Autodesk Inventor part; units mm, degrees
(part 2 of 2)
  line L170 (-11.4491, 40.8252) -> (-11.4491, 40.6608)
  line L171 (-11.4491, 40.6608) -> (-13.491, 40.6608)
  line L172 (-13.491, 40.6608) -> (-13.491, 40.8252)
  spline S328 degree 2 poles (-13.491, 40.8252) (-13.2171, 40.8252) (-13.0627, 40.9098) knots 0 0 0 1 1 1
  spline S329 degree 2 poles (-13.0627, 40.9098) (-12.9731, 40.9547) (-12.8635, 41.2087) (-12.8635, 41.5922) knots 0 0 0 1 2 2 2
  line L173 (-12.8635, 41.5922) -> (-12.8635, 45.3225)
  spline S330 degree 2 poles (-12.8635, 45.3225) (-12.8635, 46.0247) (-12.9332, 46.3435) (-13.0727, 46.458) (-13.1872, 46.458) knots 0 0 0 1 2 3 3 3
  spline S331 degree 2 poles (-13.1872, 46.458) (-13.2819, 46.458) (-13.491, 46.3883) knots 0 0 0 1 1 1
  line L174 (-13.491, 46.3883) -> (-13.5558, 46.5526)
  line L175 (-13.5558, 46.5526) -> (-12.3256, 47.0557)
  line L176 (-12.3256, 47.0557) -> (-12.1165, 47.0557)
  line L177 (-2.4844, 42.6978) -> (-4.855, 42.6978)
  line L178 (-4.855, 42.6978) -> (-5.2684, 41.7416)
  spline S332 degree 2 poles (-5.2684, 41.7416) (-5.4228, 41.383) (-5.4228, 41.2087) knots 0 0 0 1 1 1
  spline S333 degree 2 poles (-5.4228, 41.2087) (-5.4228, 41.0692) (-5.1539, 40.8551) (-4.7156, 40.8252) knots 0 0 0 1 2 2 2
  line L179 (-4.7156, 40.8252) -> (-4.7156, 40.6608)
  line L180 (-4.7156, 40.6608) -> (-6.638, 40.6608)
  line L181 (-6.638, 40.6608) -> (-6.638, 40.8252)
  spline S334 degree 2 poles (-6.638, 40.8252) (-6.2545, 40.8949) (-6.145, 40.9995) knots 0 0 0 1 1 1
  spline S335 degree 2 poles (-6.145, 40.9995) (-5.9159, 41.2186) (-5.637, 41.881) knots 0 0 0 1 1 1
  line L182 (-5.637, 41.881) -> (-3.4854, 46.8963)
  line L183 (-3.4854, 46.8963) -> (-3.3261, 46.8963)
  line L184 (-3.3261, 46.8963) -> (-1.2044, 41.8262)
  spline S336 degree 2 poles (-1.2044, 41.8262) (-0.9504, 41.2137) (-0.5321, 40.8501) (-0.1585, 40.8252) knots 0 0 0 1 2 2 2
  line L185 (-0.1585, 40.8252) -> (-0.1585, 40.6608)
  line L186 (-0.1585, 40.6608) -> (-2.5641, 40.6608)
  line L187 (-2.5641, 40.6608) -> (-2.5641, 40.8252)
  spline S337 degree 2 poles (-2.5641, 40.8252) (-2.2005, 40.8451) (-1.9415, 41.0493) (-1.9415, 41.1987) knots 0 0 0 1 2 2 2
  spline S338 degree 2 poles (-1.9415, 41.1987) (-1.9415, 41.3979) (-2.1208, 41.8262) knots 0 0 0 1 1 1
  line L188 (-2.1208, 41.8262) -> (-2.4844, 42.6978)
  line L189 (-2.6238, 43.0315) -> (-3.6498, 45.4968)
  line L190 (-3.6498, 45.4968) -> (-4.7156, 43.0315)
  line L191 (-4.7156, 43.0315) -> (-2.6238, 43.0315)
  line L192 (3.8407, 44.7796) -> (3.8407, 42.2795)
  spline S339 degree 2 poles (3.8407, 42.2795) (3.8407, 41.5722) (3.9105, 41.2535) (4.0549, 41.129) (4.1545, 41.129) knots 0 0 0 1 2 3 3 3
  spline S340 degree 2 poles (4.1545, 41.129) (4.2939, 41.129) (4.4683, 41.2037) knots 0 0 0 1 1 1
  line L193 (4.4683, 41.2037) -> (4.533, 41.0393)
  line L194 (4.533, 41.0393) -> (3.3028, 40.5363)
  line L195 (3.3028, 40.5363) -> (3.0986, 40.5363)
  line L196 (3.0986, 40.5363) -> (3.0986, 41.4079)
  spline S341 degree 2 poles (3.0986, 41.4079) (2.5657, 40.8351) (2.0129, 40.5363) (1.6992, 40.5363) knots 0 0 0 1 2 2 2
  spline S342 degree 2 poles (1.6992, 40.5363) (1.3555, 40.5363) (0.8475, 40.9348) (0.6483, 41.5673) (0.6483, 42.14) knots 0 0 0 1 2 3 3 3
  line L197 (0.6483, 42.14) -> (0.6483, 43.9778)
  spline S343 degree 2 poles (0.6483, 43.9778) (0.6483, 44.2716) (0.5238, 44.4957) (0.2748, 44.6202) (-0.049, 44.6153) knots 0 0 0 1 2 3 3 3
  line L198 (-0.049, 44.6153) -> (-0.049, 44.7796)
  line L199 (-0.049, 44.7796) -> (1.3954, 44.7796)
  line L200 (1.3954, 44.7796) -> (1.3954, 42.0255)
  spline S344 degree 2 poles (1.3954, 42.0255) (1.3954, 41.4477) (1.7938, 41.0891) (2.0777, 41.0891) knots 0 0 0 1 2 2 2
  spline S345 degree 2 poles (2.0777, 41.0891) (2.2719, 41.0891) (2.76, 41.3332) (3.0986, 41.6718) knots 0 0 0 1 2 2 2
  line L201 (3.0986, 41.6718) -> (3.0986, 44.0077)
  spline S346 degree 2 poles (3.0986, 44.0077) (3.0986, 44.3563) (2.8397, 44.6053) (2.4313, 44.6153) knots 0 0 0 1 2 2 2
  line L202 (2.4313, 44.6153) -> (2.4313, 44.7796)
  line L203 (2.4313, 44.7796) -> (3.8407, 44.7796)
  spline S347 degree 2 poles (5.9375, 42.1649) (5.559, 42.3492) (5.1555, 43.0066) (5.1555, 43.41) knots 0 0 0 1 2 2 2
  spline S348 degree 2 poles (5.1555, 43.41) (5.1555, 44.0176) (6.0769, 44.8991) (6.7991, 44.8991) knots 0 0 0 1 2 2 2
  spline S349 degree 2 poles (6.7991, 44.8991) (7.3868, 44.8991) (7.8201, 44.6103) knots 0 0 0 1 1 1
  line L204 (7.8201, 44.6103) -> (8.6916, 44.6103)
  spline S350 degree 2 poles (8.6916, 44.6103) (8.8859, 44.6103) (8.9506, 44.5904) (8.9655, 44.5605) knots 0 0 0 1 2 2 2
  spline S351 degree 2 poles (8.9655, 44.5605) (8.9905, 44.5206) (8.9905, 44.416) knots 0 0 0 1 1 1
  spline S352 degree 2 poles (8.9905, 44.416) (8.9905, 44.3015) (8.9655, 44.2567) knots 0 0 0 1 1 1
  spline S353 degree 2 poles (8.9655, 44.2567) (8.9556, 44.2318) (8.8859, 44.2069) (8.6916, 44.2069) knots 0 0 0 1 2 2 2
  line L205 (8.6916, 44.2069) -> (8.1537, 44.2069)
  spline S354 degree 2 poles (8.1537, 44.2069) (8.4077, 43.8831) (8.4077, 43.3801) knots 0 0 0 1 1 1
  spline S355 degree 2 poles (8.4077, 43.3801) (8.4077, 42.8024) (7.5262, 41.9856) (6.7841, 41.9856) knots 0 0 0 1 2 2 2
  spline S356 degree 2 poles (6.7841, 41.9856) (6.4803, 41.9856) (6.1566, 42.0753) knots 0 0 0 1 1 1
  spline S357 degree 2 poles (6.1566, 42.0753) (5.9624, 41.9059) (5.8229, 41.6519) (5.8229, 41.5623) knots 0 0 0 1 2 2 2
  spline S358 degree 2 poles (5.8229, 41.5623) (5.8229, 41.4826) (5.9723, 41.3382) (6.1865, 41.3083) knots 0 0 0 1 2 2 2
  spline S359 degree 2 poles (6.1865, 41.3083) (6.311, 41.2884) (6.819, 41.2784) knots 0 0 0 1 1 1
  spline S360 degree 2 poles (6.819, 41.2784) (7.7454, 41.2535) (8.0193, 41.2137) knots 0 0 0 1 1 1
  spline S361 degree 2 poles (8.0193, 41.2137) (8.4376, 41.1539) (8.9357, 40.6509) (8.9357, 40.2873) knots 0 0 0 1 2 2 2
  spline S362 degree 2 poles (8.9357, 40.2873) (8.9357, 39.7793) (8.4575, 39.336) knots 0 0 0 1 1 1
  spline S363 degree 2 poles (8.4575, 39.336) (7.7553, 38.6786) (6.6248, 38.6786) knots 0 0 0 1 1 1
  spline S364 degree 2 poles (6.6248, 38.6786) (5.7582, 38.6786) (5.1605, 39.0671) knots 0 0 0 1 1 1
  spline S365 degree 2 poles (5.1605, 39.0671) (4.8219, 39.2912) (4.8219, 39.5353) knots 0 0 0 1 1 1
  spline S366 degree 2 poles (4.8219, 39.5353) (4.8219, 39.6448) (4.8717, 39.7494) knots 0 0 0 1 1 1
  spline S367 degree 2 poles (4.8717, 39.7494) (4.9464, 39.9188) (5.1854, 40.2126) knots 0 0 0 1 1 1
  spline S368 degree 2 poles (5.1854, 40.2126) (5.2203, 40.2524) (5.6436, 40.6957) knots 0 0 0 1 1 1
  spline S369 degree 2 poles (5.6436, 40.6957) (5.4145, 40.8351) (5.2203, 41.0593) (5.2203, 41.1987) knots 0 0 0 1 2 2 2
  spline S370 degree 2 poles (5.2203, 41.1987) (5.2203, 41.3531) (5.4743, 41.7764) (5.9375, 42.1649) knots 0 0 0 1 2 2 2
  spline S371 degree 2 poles (5.8926, 40.6608) (5.6785, 40.4317) (5.4643, 40.0383) (5.4643, 39.8739) knots 0 0 0 1 2 2 2
  spline S372 degree 2 poles (5.4643, 39.8739) (5.4643, 39.6598) (5.7233, 39.5004) knots 0 0 0 1 1 1
  spline S373 degree 2 poles (5.7233, 39.5004) (6.1765, 39.2215) (7.0282, 39.2215) knots 0 0 0 1 1 1
  spline S374 degree 2 poles (7.0282, 39.2215) (7.835, 39.2215) (8.607, 39.7893) (8.607, 40.108) knots 0 0 0 1 2 2 2
  spline S375 degree 2 poles (8.607, 40.108) (8.607, 40.3421) (8.3779, 40.4417) knots 0 0 0 1 1 1
  spline S376 degree 2 poles (8.3779, 40.4417) (8.1438, 40.5363) (7.4515, 40.5562) knots 0 0 0 1 1 1
  spline S377 degree 2 poles (7.4515, 40.5562) (6.4355, 40.5811) (5.8926, 40.6608) knots 0 0 0 1 1 1
  spline S378 degree 2 poles (6.7194, 44.685) (6.3857, 44.685) (5.9375, 44.1571) (5.9375, 43.6092) knots 0 0 0 1 2 2 2
  spline S379 degree 2 poles (5.9375, 43.6092) (5.9375, 42.897) (6.2413, 42.5086) knots 0 0 0 1 1 1
  spline S380 degree 2 poles (6.2413, 42.5086) (6.4754, 42.2097) (6.8389, 42.2097) knots 0 0 0 1 1 1
  spline S381 degree 2 poles (6.8389, 42.2097) (7.1776, 42.2097) (7.6208, 42.7227) (7.6208, 43.2706) knots 0 0 0 1 2 2 2
  spline S382 degree 2 poles (7.6208, 43.2706) (7.6208, 43.9828) (7.3121, 44.3862) knots 0 0 0 1 1 1
  spline S383 degree 2 poles (7.3121, 44.3862) (7.083, 44.685) (6.7194, 44.685) knots 0 0 0 1 1 1
  line L206 (15.6791, 41.8312) -> (15.2508, 40.6608)
  line L207 (15.2508, 40.6608) -> (11.655, 40.6608)
  line L208 (11.655, 40.6608) -> (11.655, 40.8252)
  spline S384 degree 2 poles (11.655, 40.8252) (13.2437, 42.2745) (14.5386, 44.1073) (14.5386, 44.8693) knots 0 0 0 1 2 2 2
  spline S385 degree 2 poles (14.5386, 44.8693) (14.5386, 45.447) (13.8264, 46.194) (13.3334, 46.194) knots 0 0 0 1 2 2 2
  spline S386 degree 2 poles (13.3334, 46.194) (12.8801, 46.194) (12.1679, 45.6661) (11.9936, 45.1581) knots 0 0 0 1 2 2 2
  line L209 (11.9936, 45.1581) -> (11.8293, 45.1581)
  spline S387 degree 2 poles (11.8293, 45.1581) (11.9438, 45.9898) (12.8702, 46.8813) (13.5674, 46.8813) knots 0 0 0 1 2 2 2
  spline S388 degree 2 poles (13.5674, 46.8813) (14.3095, 46.8813) (15.3056, 45.9301) (15.3056, 45.2826) knots 0 0 0 1 2 2 2
  spline S389 degree 2 poles (15.3056, 45.2826) (15.3056, 44.8195) (15.0914, 44.3563) knots 0 0 0 1 1 1
  spline S390 degree 2 poles (15.0914, 44.3563) (14.7577, 43.6291) (14.0107, 42.8124) knots 0 0 0 1 1 1
  spline S391 degree 2 poles (14.0107, 42.8124) (12.8901, 41.5922) (12.6112, 41.3382) knots 0 0 0 1 1 1
  line L210 (12.6112, 41.3382) -> (14.2049, 41.3382)
  spline S392 degree 2 poles (14.2049, 41.3382) (14.693, 41.3382) (15.0815, 41.4079) (15.3952, 41.632) (15.5148, 41.8312) knots 0 0 0 1 2 3 3 3
  line L211 (15.5148, 41.8312) -> (15.6791, 41.8312)
  spline S393 degree 2 poles (16.3963, 43.674) (16.3963, 44.7149) (17.0238, 46.2189) (17.5468, 46.5875) knots 0 0 0 1 2 2 2
  spline S394 degree 2 poles (17.5468, 46.5875) (17.9502, 46.8813) (18.3835, 46.8813) knots 0 0 0 1 1 1
  spline S395 degree 2 poles (18.3835, 46.8813) (19.0857, 46.8813) (19.6435, 46.1691) knots 0 0 0 1 1 1
  spline S396 degree 2 poles (19.6435, 46.1691) (20.3408, 45.2826) (20.3408, 43.7686) knots 0 0 0 1 1 1
  spline S397 degree 2 poles (20.3408, 43.7686) (20.3408, 42.7078) (19.7282, 41.2236) (18.7819, 40.5562) (18.3386, 40.5562) knots 0 0 0 1 2 3 3 3
  spline S398 degree 2 poles (18.3386, 40.5562) (17.4671, 40.5562) (16.8844, 41.5872) knots 0 0 0 1 1 1
  spline S399 degree 2 poles (16.8844, 41.5872) (16.3963, 42.4538) (16.3963, 43.674) knots 0 0 0 1 1 1
  spline S400 degree 2 poles (17.2778, 43.5594) (17.2778, 42.3044) (17.5866, 41.5075) knots 0 0 0 1 1 1
  spline S401 degree 2 poles (17.5866, 41.5075) (17.8456, 40.8401) (18.3536, 40.8401) knots 0 0 0 1 1 1
  spline S402 degree 2 poles (18.3536, 40.8401) (18.5976, 40.8401) (19.1156, 41.2734) (19.2501, 41.7864) knots 0 0 0 1 2 2 2
  spline S403 degree 2 poles (19.2501, 41.7864) (19.4592, 42.5584) (19.4592, 43.9628) knots 0 0 0 1 1 1
  spline S404 degree 2 poles (19.4592, 43.9628) (19.4592, 45.0087) (19.2451, 45.701) knots 0 0 0 1 1 1
  spline S405 degree 2 poles (19.2451, 45.701) (19.0807, 46.2189) (18.8267, 46.4331) knots 0 0 0 1 1 1
  spline S406 degree 2 poles (18.8267, 46.4331) (18.6425, 46.5825) (18.3785, 46.5825) knots 0 0 0 1 1 1
  spline S407 degree 2 poles (18.3785, 46.5825) (18.0747, 46.5825) (17.8356, 46.3086) knots 0 0 0 1 1 1
  spline S408 degree 2 poles (17.8356, 46.3086) (17.5119, 45.9351) (17.2778, 44.3364) (17.2778, 43.5594) knots 0 0 0 1 2 2 2
  line L212 (24.8928, 41.8312) -> (24.4645, 40.6608)
  line L213 (24.4645, 40.6608) -> (20.8687, 40.6608)
  line L214 (20.8687, 40.6608) -> (20.8687, 40.8252)
  spline S409 degree 2 poles (20.8687, 40.8252) (22.4574, 42.2745) (23.7523, 44.1073) (23.7523, 44.8693) knots 0 0 0 1 2 2 2
  spline S410 degree 2 poles (23.7523, 44.8693) (23.7523, 45.447) (23.0401, 46.194) (22.5471, 46.194) knots 0 0 0 1 2 2 2
  spline S411 degree 2 poles (22.5471, 46.194) (22.0939, 46.194) (21.3817, 45.6661) (21.2074, 45.1581) knots 0 0 0 1 2 2 2
  line L215 (21.2074, 45.1581) -> (21.043, 45.1581)
  spline S412 degree 2 poles (21.043, 45.1581) (21.1575, 45.9898) (22.0839, 46.8813) (22.7812, 46.8813) knots 0 0 0 1 2 2 2
  spline S413 degree 2 poles (22.7812, 46.8813) (23.5232, 46.8813) (24.5193, 45.9301) (24.5193, 45.2826) knots 0 0 0 1 2 2 2
  spline S414 degree 2 poles (24.5193, 45.2826) (24.5193, 44.8195) (24.3052, 44.3563) knots 0 0 0 1 1 1
  spline S415 degree 2 poles (24.3052, 44.3563) (23.9715, 43.6291) (23.2244, 42.8124) knots 0 0 0 1 1 1
  spline S416 degree 2 poles (23.2244, 42.8124) (22.1038, 41.5922) (21.8249, 41.3382) knots 0 0 0 1 1 1
  line L216 (21.8249, 41.3382) -> (23.4186, 41.3382)
  spline S417 degree 2 poles (23.4186, 41.3382) (23.9067, 41.3382) (24.2952, 41.4079) (24.609, 41.632) (24.7285, 41.8312) knots 0 0 0 1 2 3 3 3
  line L217 (24.7285, 41.8312) -> (24.8928, 41.8312)
  line L218 (29.2756, 46.7568) -> (28.927, 45.9948)
  line L219 (28.927, 45.9948) -> (27.0942, 45.9948)
  line L220 (27.0942, 45.9948) -> (26.6908, 45.178)
  spline S418 degree 2 poles (26.6908, 45.178) (27.8811, 45.0037) (28.5783, 44.2915) knots 0 0 0 1 1 1
  spline S419 degree 2 poles (28.5783, 44.2915) (29.176, 43.6789) (29.176, 42.8522) knots 0 0 0 1 1 1
  spline S420 degree 2 poles (29.176, 42.8522) (29.176, 42.3741) (28.7825, 41.5523) (28.1899, 40.9796) (27.8263, 40.8053) knots 0 0 0 1 2 3 3 3
  spline S421 degree 2 poles (27.8263, 40.8053) (27.3083, 40.5562) (26.7655, 40.5562) knots 0 0 0 1 1 1
  spline S422 degree 2 poles (26.7655, 40.5562) (26.2126, 40.5562) (25.7146, 40.9298) (25.7146, 41.1539) knots 0 0 0 1 2 2 2
  spline S423 degree 2 poles (25.7146, 41.1539) (25.7146, 41.2784) (25.9188, 41.4726) (26.0782, 41.4726) knots 0 0 0 1 2 2 2
  spline S424 degree 2 poles (26.0782, 41.4726) (26.1927, 41.4726) (26.372, 41.3979) (26.5812, 41.2485) knots 0 0 0 1 2 2 2
  spline S425 degree 2 poles (26.5812, 41.2485) (26.9199, 41.0194) (27.2685, 41.0144) knots 0 0 0 1 1 1
  spline S426 degree 2 poles (27.2685, 41.0144) (27.7914, 41.0144) (28.5933, 41.8113) (28.5933, 42.384) knots 0 0 0 1 2 2 2
  spline S427 degree 2 poles (28.5933, 42.384) (28.5933, 42.9369) (27.8811, 43.8981) (27.2535, 44.1571) knots 0 0 0 1 2 2 2
  spline S428 degree 2 poles (27.2535, 44.1571) (26.7655, 44.3613) (25.9188, 44.3911) knots 0 0 0 1 1 1
  line L221 (25.9188, 44.3911) -> (27.0892, 46.7568)
  line L222 (27.0892, 46.7568) -> (29.2756, 46.7568)
  point P0 (0, 0)
  dimension "d0" = 178.9
  constraints: 2 other
emboss "Emboss1" sketch "Sketch6" operation cut depth 1.5 direction (-1, 0, 0)
ref_plane "Work Plane1" through (-1, 0, 0) normal (-1, 0, 0) x (0, 0, 1)
sketch "Sketch7" plane through (-1, 0, 0) normal (-1, 0, 0) x (0, 0, 1)
  arc A0 (53.877, -77.183) -> (48.877, -77.183) centre (51.377, -77.183) ccw
  arc A1 (-48.877, -77.183) -> (-53.877, -77.183) centre (-51.377, -77.183) ccw
  line L0 (54.5, -89.45) -> (-54.5, -89.45) projected
  line L1 (54.5, 89.45) -> (54.5, -89.45) projected
  line L2 (-54.5, -89.45) -> (-54.5, 89.45) projected
  line L3 (53.877, -77.183) -> (48.877, -77.183)
  line L4 (-48.877, -77.183) -> (-53.877, -77.183)
  point P0 (0, 0)
  dimension "d22" = 12.267
  dimension "d23" = 3.123
  dimension "d24" = 12.267
  dimension "d25" = 3.123
  dimension "d26" = 5
  dimension "d27" = 5
  constraints: 4 end point, 4 point on circle, 2 centre point, 2 point on line, 1 horizontal
  measures "d22" distance from line of L0 A0.centre
  measures "d23" distance from line of A0.centre L1
  measures "d24" distance from line of L0 A1.centre
  measures "d25" distance from line of L2 A1.centre
  measures "d26" diameter of A0
  measures "d27" diameter of A1
revolve "Revolution1" cut sketch "Sketch7" angle 360 about axis through (-1, -77.183, -48.877) along (0, 0, -1)
body "Solid1"
